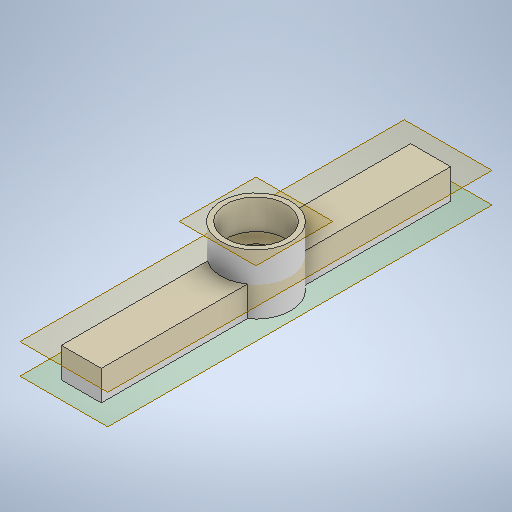
# Autodesk Inventor part: wing1
Saved by Autodesk Inventor 2025.2 (Build 292293000, 293)
## iProperties
Created: 2024-12-15
Part Number: wing1
Material: 一般
Document SubType Name: Modeling
Designer: mahhy
Density: 1 g/cm^3
Appearance: 既定
Author: mahhy
Autodesk Inventor part; units mm, degrees
ref_plane "YZ Plane" through (0, 0, 0) normal (1, 0, 0) x (0, 1, 0)
ref_plane "XZ Plane" through (0, 0, 0) normal (0, 1, 0) x (-1, 0, 0)
ref_plane "XY Plane" through (0, 0, 0) normal (0, 0, 1) x (1, 0, 0)
sketch "スケッチ1" plane through (0, 0, 0) normal (0, 1, 0) x (-1, 0, 0)
  line L0 (0, 0) -> (4, 0)
  line L1 (4, 0) -> (4, -35)
  line L2 (4, -35) -> (0, -35)
  line L3 (0, -35) -> (0, 0)
  circle A0 centre (2, -17.5) radius 3.5
  point P0 (2, 0)
  point P1 (2, -35)
  point P2 (4, -20.3723)
  point P3 (4, -14.6277)
  point P4 (0, -14.6277)
  point P5 (0, -20.3723)
  dimension "d0" = 4
  dimension "d1" = 35
  dimension "d3" = 7
  constraints: 8 end point, 2 midpoint, 2 parallel, 1 centre point, 1 horizontal, 1 perpendicular
  measures "d0" distance of L1.end L2.end
  measures "d1" distance of L0.end L1.end
  measures "d3" diameter of A0
extrude "押し出し1" add sketch "スケッチ1" along normal blind 3
ref_plane "作業平面1" through (0, 3, 0) normal (0, 1, 0) x (1, 0, 0)
sketch "スケッチ2" plane through (0, 3, 0) normal (0, 1, 0) x (1, 0, 0)
  line L0 (-4, 0) -> (0, 0) projected
  line L1 (0, 35) -> (-4, 35) projected
  arc A0 (0, 14.6277) -> (0, 20.3723) centre (-2, 17.5) ccw projected
  circle A1 centre (-2, 17.5) radius 3.5
  point P0 (-2, 0)
  point P1 (-2, 35)
  dimension "d7" = 7
  constraints: 2 coincident, 2 midpoint, 1 centre point
  measures "d7" diameter of A1
extrude "押し出し2" add sketch "スケッチ2" along normal blind 3
ref_plane "作業平面2" through (0, 0, 0) normal (0, -1, 0) x (1, 0, 0)
sketch "スケッチ3" plane through (0, 0, 0) normal (0, -1, 0) x (1, 0, 0)
  arc A0 (-4, -14.6277) -> (-4, -20.3723) centre (-2, -17.5) ccw projected
  circle A1 centre (-2, -17.5) radius 1.5
  point P0 (0, 0)
  dimension "d11" = 3
  constraints: 1 centre point, 1 coincident
  measures "d11" diameter of A1
extrude "押し出し3" cut sketch "スケッチ3" against normal through all
ref_plane "作業平面3" through (-2, 6, -17.5) normal (0, 1, 0) x (1, 0, 0)
sketch "スケッチ4" plane through (-2, 6, -17.5) normal (0, 1, 0) x (1, 0, 0)
  circle A0 centre (0, 0) radius 1.5 projected
  circle A1 centre (0, 0) radius 3
  point P0 (2, -17.5)
  dimension "d15" = 6
  constraints: 1 centre point, 1 coincident
  measures "d15" diameter of A1
extrude "押し出し4" cut sketch "スケッチ4" against normal blind 3
